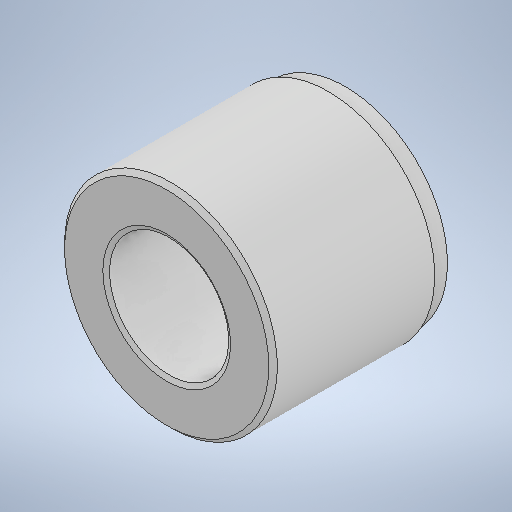
# Autodesk Inventor part: 26-10-209_ZI01
Saved by Autodesk Inventor 2025.2 (Build 292293000, 293)
## iProperties
Created: 2025-01-09
Part Number: 26-10-209_ZI01
Material: Generic
Document SubType Name: Modeling
Designer: Zvonko.Gabric
Density: 1 g/cm^3
Appearance: Default
Author: Zvonko.Gabric
Autodesk Inventor part; units mm, degrees
ref_plane "YZ Plane" through (0, 0, 0) normal (1, 0, 0) x (0, 1, 0)
ref_plane "XZ Plane" through (0, 0, 0) normal (0, 1, 0) x (-1, 0, 0)
ref_plane "XY Plane" through (0, 0, 0) normal (0, 0, 1) x (1, 0, 0)
sketch "Sketch1" plane through (0, 0, 0) normal (0, 1, 0) x (-1, 0, 0)
  line L0 (0, 0) -> (0, -21) construction
  line L1 (7, -21) -> (12, -21)
  line L2 (12, -21) -> (12, -19)
  line L3 (12, -19) -> (12.5, -19)
  line L4 (12.5, -19) -> (12.5, -0.5)
  line L5 (12.5, -0.5) -> (12, 0)
  line L6 (12, 0) -> (8.2431, 0)
  line L7 (7, -0.289) -> (7, -21)
  line L8 (8.2431, 0) -> (7.5, 0)
  line L9 (7, -0.289) -> (7.5, 0)
  point P0 (12, -20)
  dimension "d0" = 21
  dimension "d2" = 12
  dimension "d3" = 2
  dimension "d4" = 18.5
  dimension "d5" = 21
  dimension "d6" = 0
  dimension "d7" = 7.5
  dimension "d8" = 0.289
  dimension "d9" = 12.5
  dimension "d10" = 5.5
  constraints: 20 end point, 4 perpendicular, 1 horizontal, 1 midpoint, 1 parallel, 1 point on line, 1 vertical
  measures "d0" distance of L0.start L0.end
  measures "d2" distance from line of L0 point (12, -20)
  measures "d3" distance of L1.end L2.end
  measures "d4" distance of L3.end L4.end
  measures "d5" distance between parallel lines of L6 L1
  measures "d6" vertical distance of L0.start L8.end
  measures "d7" distance from line of L8.end L0
  measures "d8" vertical distance of L8.end L7.start
  measures "d9" distance between parallel lines of L0 L4
  measures "d10" distance between parallel lines of L4 L7
revolve "Revolution1" add sketch "Sketch1" angle 360 about axis through (0, 0, 0) along (0, 0, -1)
body "Solid1"
